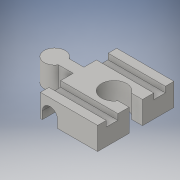
# Autodesk Inventor part: traintrack
Saved by Autodesk Inventor 2016 (Build 200138000, 138)
## iProperties
Created: 2015-08-30
Part Number: traintrack
Material: Generic
Document SubType Name: Modeling
Designer: adam
Density: 1 g/cm^3
Appearance: Default
Author: adam
Autodesk Inventor part; units mm, degrees
ref_plane "YZ Plane" through (0, 0, 0) normal (1, 0, 0) x (0, 1, 0)
ref_plane "XZ Plane" through (0, 0, 0) normal (0, 1, 0) x (-1, 0, 0)
ref_plane "XY Plane" through (0, 0, 0) normal (0, 0, 1) x (1, 0, 0)
sketch "Sketch1" plane through (0, 0, 0) normal (0, 1, 0) x (-1, 0, 0)
  line L0 (9.5606, 37.6724) -> (-20.4394, 37.6724)
  line L1 (-20.4394, -2.3276) -> (9.5606, -2.3276)
  line L2 (17.3267, 20.4724) -> (9.5606, 20.4724)
  line L3 (9.5606, 14.8724) -> (17.3267, 14.8724)
  arc A0 (17.3267, 14.8724) -> (17.3267, 20.4724) centre (22.0606, 17.6724) ccw
  line L4 (9.5606, -2.3276) -> (9.5606, 14.8724)
  line L5 (9.5606, 20.4724) -> (9.5606, 37.6724)
  arc A1 (-14.6894, 14.1724) -> (-14.6894, 21.1724) centre (-9.0644, 17.6724) ccw
  line L6 (-14.6894, 21.1724) -> (-20.4394, 21.1724)
  line L7 (-14.6894, 14.1724) -> (-20.4394, 14.1724)
  line L8 (-20.4394, 37.6724) -> (-20.4394, 21.1724)
  line L9 (-20.4394, 14.1724) -> (-20.4394, -2.3276)
  point P0 (0, 0)
  dimension "d0" = 30
  dimension "d1" = 40
  dimension "d2" = 17.2
  dimension "d5" = 17.2
  dimension "d10" = 12.5
  dimension "d12" = 7.7661
  dimension "d17" = 13.25
  dimension "d18" = 20
  dimension "d19" = 16.5
  dimension "d20" = 16.5
  constraints: 20 end point, 6 parallel, 6 perpendicular, 4 point on circle, 2 centre point, 2 horizontal, 1 collinear
  measures "d0" distance of L1.end L1.start
  measures "d1" distance of L0.end L1.start
  measures "d2" distance between parallel lines of L1 L3
  measures "d5" distance between parallel lines of L2 L0
  measures "d10" distance from line of L5 A0.centre
  measures "d12" distance of L3.start L3.end
  measures "d17" diameter of A1
  measures "d18" distance from line of L0 A1.centre
  measures "d19" distance between parallel lines of L0 L6
  measures "d20" distance between parallel lines of L1 L7
extrude "Extrusion1" add sketch "Sketch1" along normal blind 11.9
sketch "Sketch2" plane through (0, 11.9, 0) normal (0, 1, 0) x (1, 0, 0)
  line L0 (-9.5606, -20.4724) -> (-9.5606, -37.6724) projected
  line L1 (-9.5606, -33.1724) -> (20.4769, -33.1724)
  line L2 (20.4769, -33.1724) -> (20.4769, -27.0724)
  line L3 (20.4769, -27.0724) -> (-9.5606, -27.0724)
  line L4 (-9.5606, -27.0724) -> (-9.5606, -33.1724)
  line L5 (-9.5606, -37.6724) -> (20.4394, -37.6724) projected
  line L6 (-9.5606, -8.2724) -> (20.4769, -8.2724)
  line L7 (20.4769, -8.2724) -> (20.4769, -2.1724)
  line L8 (20.4769, -2.1724) -> (-9.5606, -2.1724)
  line L9 (-9.5606, -2.1724) -> (-9.5606, -8.2724)
  line L10 (20.4394, 2.3276) -> (-9.5606, 2.3276) projected
  line L11 (-9.5606, 2.3276) -> (-9.5606, -14.8724) projected
  point P0 (0, 0)
  dimension "d24" = 6.1
  dimension "d25" = 4.5
  dimension "d26" = 6.1
  dimension "d27" = 4.5
  dimension "d35" = 0
  constraints: 16 end point, 4 parallel, 2 horizontal, 2 perpendicular, 1 point on line
  measures "d24" distance between parallel lines of L3 L1
  measures "d25" distance between parallel lines of L5 L1
  measures "d26" distance between parallel lines of L8 L6
  measures "d27" distance between parallel lines of L10 L8
  measures "d35" distance between parallel lines of L11 L9
extrude "Extrusion2" cut sketch "Sketch2" against normal blind 3
sketch "Sketch3" plane through (20.4394, 0, -2.3276) normal (0, 0, -1) x (-1, 0, 0)
  line L0 (21, 0) -> (29, 0)
  line L1 (29, 0) -> (29, 4)
  line L2 (21, 4) -> (21, 0)
  arc A0 (29, 4) -> (21, 4) centre (25, 4) ccw
  line L3 (30, 0) -> (30, 11.9) projected
  point P0 (20.4394, 0)
  dimension "d34" = 9
  constraints: 6 end point, 2 point on circle, 2 tangent, 1 centre point, 1 horizontal, 1 parallel, 1 perpendicular
  measures "d34" distance between parallel lines of L3 L2
extrude "Extrusion3" cut sketch "Sketch3" against normal through all
body "Solid1"
